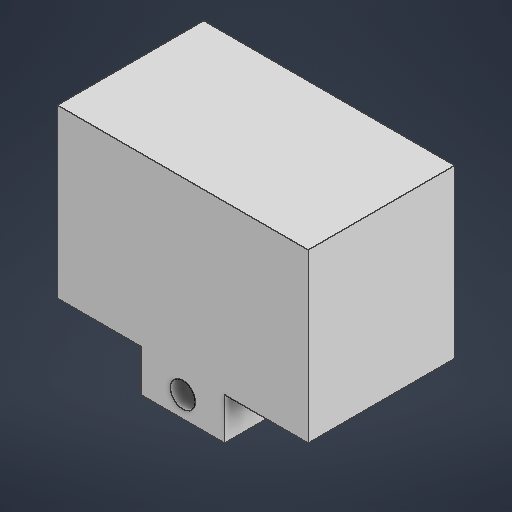
# Autodesk Inventor part: haraketli_cene
Saved by Autodesk Inventor 2025.4 (Build 294407000, 407)
## iProperties
Created: 2026-06-17
Part Number: haraketli_cene
Material: Generic
Document SubType Name: Modeling
Designer: yigithan
Density: 1 g/cm^3
Appearance: Default
Author: yigithan
Autodesk Inventor part; units mm, degrees
ref_plane "YZ Plane" through (0, 0, 0) normal (1, 0, 0) x (0, 1, 0)
ref_plane "XZ Plane" through (0, 0, 0) normal (0, 1, 0) x (-1, 0, 0)
ref_plane "XY Plane" through (0, 0, 0) normal (0, 0, 1) x (1, 0, 0)
sketch "Sketch1" plane through (0, 0, 0) normal (0, 0, 1) x (1, 0, 0)
  line L0 (0, 10) -> (0, 50)
  line L1 (0, 50) -> (60, 50)
  line L2 (60, 50) -> (60, 10)
  line L3 (60, 10) -> (40, 10)
  line L4 (40, 10) -> (40, 0)
  line L5 (40, 0) -> (20, 0)
  line L6 (20, 0) -> (20, 10)
  line L7 (20, 10) -> (0, 10)
  point P0 (0, 0)
  dimension "d0" = 40
  dimension "d1" = 60
  dimension "d2" = 20
  dimension "d3" = 20
  constraints: 16 end point, 6 perpendicular, 1 horizontal, 1 point on line, 1 vertical
  measures "d0" distance of L0.start L0.end
  measures "d1" distance of L0.end L1.end
  measures "d2" distance of L2.end L3.end
  measures "d3" distance of L4.end L5.end
extrude "Extrusion1" add sketch "Sketch1" along normal blind 35
sketch "Sketch2" plane through (0, 0, 35) normal (0, 0, 1) x (1, 0, 0)
  circle A0 centre (30, 5) radius 3
  line L0 (20, 10) -> (20, 0) projected
  line L1 (20, 0) -> (40, 0) projected
  point P0 (0, 0)
  point P1 (20, 5)
  point P2 (30, 0)
  dimension "d6" = 6
  dimension "d7" = 10
  dimension "d8" = 5
  constraints: 2 midpoint, 1 centre point
  measures "d6" diameter of A0
  measures "d7" distance of A0.centre point (20, 5)
  measures "d8" distance of point (30, 0) A0.centre
extrude "Extrusion2" cut sketch "Sketch2" against normal blind 35
body "Solid1"
